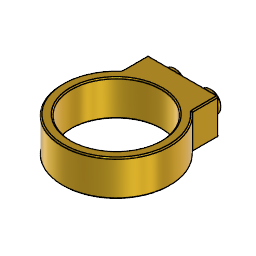
Brick Ring (Autodesk Fusion 360 design; units mm, degrees)
part number: 2026-06-10-18-29-48-389
Autodesk Fusion 360 part; units mm, degrees
note: some values were not read from the file. Set by a fixed rule: which sketch regions a step uses.
sketch "Sketch1" plane through (0, 0, 0) normal (0, 0, 1) x (1, 0, 0)
  circle A0 centre (0, 0) radius 12
  line L0 (7.9, 15) -> (-7.9, 15)
  line L1 (-7.9, 15) -> (-7.9, 9)
  line L2 (-7.9, 9) -> (7.9, 9)
  line L3 (7.9, 9) -> (7.9, 15)
  line L4 (7.9, 15) -> (-7.9, 9) construction
  line L5 (-7.9, 15) -> (7.9, 9) construction
  point P0 (0, 12)
  dimension "d1" = 24
  dimension "d2" = 15.8
  dimension "d3" = 6
  constraint coincident A0.centre origin
  constraint horizontal L0
  constraint perpendicular L0 L1
  constraint parallel L0 L2
  constraint parallel L1 L3
  constraint coincident L4 P0
  constraint coincident L5 P0
  constraint coincident A0 P0
  constraint vertical A0.centre P0
  measures "d1" diameter of A0
  measures "d2" distance of L0.start L0.end
  measures "d3" distance of L0.end L1.end
extrude "Extrude1" add sketch "Sketch1" along normal blind 8
sketch "Sketch2" plane through (0, 0, 8) normal (0, 0, 1) x (-1, 0, 0)
  arc A0 (7.9, -9.0327) -> (-7.9, -9.0327) centre (0, 0) ccw
  line L0 (-7.9, -9.0327) -> (-7.9, -15)
  line L1 (-7.9, -15) -> (7.9, -15)
  line L2 (7.9, -15) -> (7.9, -9.0327)
  circle A1 centre (0, 0) radius 10
  dimension "d6" = 20
  constraint concentric A0 A1
  measures "d6" diameter of A1
extrude "Extrude2" cut sketch "Sketch2" against normal blind 8 contours A1
sketch "Sketch3" plane through (0, 15, 0) normal (0, 1, 0) x (-1, 0, 0)
  line L0 (-7.9, 0) -> (7.9, 0)
  line L1 (7.9, 0) -> (7.9, 8)
  line L2 (7.9, 8) -> (-7.9, 8)
  line L3 (-7.9, 8) -> (-7.9, 0)
  circle A0 centre (-4, 4) radius 2.425
  circle A1 centre (4, 4) radius 2.425
  dimension "d9" = 8
  dimension "d10" = 4.85
  dimension "d11" = 4
  dimension "d12" = 4
  constraint equal A0 A1
  constraint horizontal A0.centre A1.centre
  measures "d9" distance of A0.centre A1.centre
  measures "d10" diameter of A1
  measures "d11" horizontal distance of origin A0.centre
  measures "d12" distance of L2 A0.centre
extrude "Extrude3" add sketch "Sketch3" along normal blind 2.25 draft -2 contours A0 | A1
fillet "Fillet1" radius 0.25 18 edges at (0, -12, 8) (7.9, 12.0164, 8) (9.3233, -3.6162, 8) (6.1876, 17.25, 4.8485) (0, 15, 8) (6.2609, 15, 4.8769) (-1.8124, 17.25, 4.8485) (9.3233, 3.6162, 0) (-1.7391, 15, 4.8769) (0, 15, 0) (-7.9, 12.0164, 0) (-7.9, 9.0327, 4) (-7.9, 12.0164, 8) (-7.9, 15, 4) (7.9, 9.0327, 4) (0, -12, 0) (7.9, 12.0164, 0) (7.9, 15, 4) 11 faces at (3.3149, 17.25, 4.5664) (1.1535, 15, 7.4547) (-7.9, 13.0109, 2.6667) (0.2491, 13.324, 8) (-3.1204, 15.5, 1.7589) (-9.9503, 0.9957, 2.6667) (-3.826, 17.25, 4.7625) (7.9, 11.0218, 2.6667) (1.8309, 15.5, 2.9554) (0.2491, 13.324, 0) (-8.7451, 8.2173, 5.3333)
